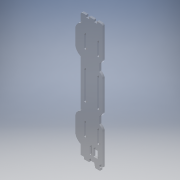
# Autodesk Inventor part: Left_wall
Saved by Autodesk Inventor 2016 (Build 200138000, 138)
## iProperties
Created: 2015-06-19
Part Number: Left_wall
Material: Generic
Document SubType Name: Modeling
Designer: Openlab
Density: 1 g/cm^3
Appearance: Polycarbonate - Clear
Author: Openlab
Autodesk Inventor part; units mm, degrees
ref_plane "YZ Plane" through (0, 0, 0) normal (1, 0, 0) x (0, 1, 0)
ref_plane "XZ Plane" through (0, 0, 0) normal (0, 1, 0) x (-1, 0, 0)
ref_plane "XY Plane" through (0, 0, 0) normal (0, 0, 1) x (1, 0, 0)
sketch "Sketch1" plane through (0, 0, 0) normal (0, 1, 0) x (-1, 0, 0)
  line L0 (26.5, -25) -> (23.5, -25)
  line L1 (26.5, -43) -> (23.5, -43)
  line L2 (26.5, -68) -> (23.5, -68)
  line L3 (26.5, -108) -> (23.5, -108)
  line L4 (8, -68) -> (5, -68)
  line L5 (8, -108) -> (5, -108)
  line L6 (8, -43) -> (5, -43)
  line L7 (8, -25) -> (5, -25)
  line L8 (23.5, -108) -> (23.5, -68)
  line L9 (23.5, -43) -> (23.5, -25)
  line L10 (8, -108) -> (8, -68)
  line L11 (8, -43) -> (8, -25)
  line L12 (8, -151) -> (8, -133)
  line L13 (26.5, -133) -> (23.5, -133)
  line L14 (8, -133) -> (5, -133)
  line L15 (23.5, -133) -> (23.5, -151)
  line L16 (23.5, -151) -> (26.5, -151)
  line L17 (5, -151) -> (8, -151)
  line L18 (18.5, -159) -> (16.7, -159)
  line L19 (16.7, -159) -> (16.7, -169)
  line L20 (16.7, -169) -> (18.5, -169)
  line L21 (18.5, -169) -> (18.5, -159)
  line L22 (15.75, -82) -> (15.75, -115) construction
  line L23 (13.2, -159) -> (7.2, -159)
  line L24 (7.2, -159) -> (7.2, -169)
  line L25 (7.2, -169) -> (13.2, -169)
  line L26 (13.2, -169) -> (13.2, -159)
  line L27 (26.5, -25) -> (26.5, -43)
  line L28 (26.5, -68) -> (26.5, -108)
  line L29 (26.5, -133) -> (26.5, -151)
  line L30 (5, -151) -> (5, -133)
  line L31 (5, -108) -> (5, -68)
  line L32 (5, -43) -> (5, -25)
  line L33 (12.25, -3) -> (8, -3)
  line L34 (19.25, -3) -> (19.25, 0)
  line L35 (19.25, 0) -> (12.25, 0)
  line L36 (12.25, 0) -> (12.25, -3)
  line L37 (19.25, -3) -> (23.5, -3)
  line L38 (5, -176) -> (5, -179)
  line L39 (12, -176) -> (19.5, -176)
  line L40 (19.5, -176) -> (19.5, -179)
  line L41 (19.5, -179) -> (26.2897, -179)
  line L42 (26.5, -176) -> (31.5, -176)
  line L43 (5, -179) -> (3.875, -179)
  line L44 (23.5, -3) -> (23.5, 0)
  line L45 (23.5, 0) -> (28.5, 0)
  line L46 (8, -3) -> (8, 0)
  line L47 (8, 0) -> (3, 0)
  line L48 (3.5, -180) -> (3.5, -181.5)
  line L49 (4, -182) -> (10.5533, -182)
  arc A0 (3.5, -181.5) -> (4, -182) centre (4, -181.5) ccw
  arc A1 (26.2897, -179) -> (26.5, -176) centre (5, -176) ccw
  arc A2 (5, -125.5838) -> (0, -133) centre (8, -133) ccw
  arc A3 (5, -60.5838) -> (0, -68) centre (8, -68) ccw
  line L50 (5, -50.4162) -> (5, -60.5838)
  line L51 (5, -115.4162) -> (5, -125.5838)
  line L52 (19.5, -120.5) -> (13.2, -120.5) construction
  arc A4 (0, -108) -> (5, -115.4162) centre (8, -108) ccw
  line L53 (0, -176) -> (0, -133)
  arc A5 (0, -43) -> (5, -50.4162) centre (8, -43) ccw
  line L54 (0, -108) -> (0, -68)
  line L55 (0, -43) -> (0, -3)
  arc A6 (31.5, -54.4564) -> (39, -43) centre (26.5, -43) ccw
  line L56 (39, -25) -> (39, -43)
  arc A7 (39, -25) -> (31.5, -13.5436) centre (26.5, -25) ccw
  line L57 (31.5, -3) -> (31.5, -13.5436)
  arc A8 (39, -133) -> (31.5, -121.5436) centre (26.5, -133) ccw
  line L58 (39, -151) -> (39, -133)
  arc A9 (31.5, -162.4564) -> (39, -151) centre (26.5, -151) ccw
  line L59 (31.5, -54.4564) -> (31.5, -121.5436)
  line L60 (31.5, -162.4564) -> (31.5, -176)
  line L61 (5, -176) -> (0, -176)
  line L62 (3.5, -180) -> (3.875, -179)
  line L63 (12, -176) -> (10.5533, -182)
  arc A10 (31.5, -3) -> (28.5, 0) centre (28.5, -3) ccw
  arc A11 (3, 0) -> (0, -3) centre (3, -3) ccw
  point P0 (0, 0)
  point P1 (3.5, -179)
  dimension "d7" = 18
  dimension "d8" = 25
  dimension "d9" = 40
  dimension "d39" = 18
  dimension "d43" = 1.8
  dimension "d45" = 10
  dimension "d51" = 3.5
  dimension "d52" = 6
  dimension "d56" = 3
  dimension "d61" = 25
  dimension "d62" = 15.5
  dimension "d63" = 22
  dimension "d64" = 25
  dimension "d65" = 7
  dimension "d74" = 173
  dimension "d75" = 15.5
  dimension "d80" = 3
  dimension "d81" = 1.5
  dimension "d82" = 7
  dimension "d85" = 7
  dimension "d90" = 5
  dimension "d92" = 25
  dimension "d94" = 13
  dimension "d97" = 1
  dimension "d98" = 0.5
  dimension "d100" = 7.5
  dimension "d101" = 7
  dimension "d102" = 5
  dimension "d103" = 7
  dimension "d104" = 6
  constraints: 129 end point, 24 collinear, 24 point on circle, 20 tangent, 15 point on line, 12 centre point, 10 perpendicular, 8 vertical, 7 coincident, 7 equal length, 5 horizontal, 5 parallel, 4 equal radius, 5 other
  measures "d7" distance between parallel lines of L1 L0
  measures "d8" distance between parallel lines of L2 L1
  measures "d9" distance between parallel lines of L3 L2
  measures "d39" distance of L13.end L15.end
  measures "d43" distance of L18.start L18.end
  measures "d45" distance of L20.end L18.start
  measures "d51" distance between parallel lines of L19 L26
  measures "d52" distance of L23.start L23.end
  measures "d56" distance of L0.start L0.end
  measures "d61" distance between parallel lines of L3 L13
  measures "d62" distance between parallel lines of L10 L8
  measures "d63" distance between parallel lines of L37 L0
  measures "d64" distance between parallel lines of L16 L42
  measures "d65" distance of L34.end L35.end
  measures "d74" distance between parallel lines of L42 L37
  measures "d75" distance between parallel lines of L46 L44
  measures "d80" distance between parallel lines of L49 L43
  measures "d81" distance between parallel lines of L48 L38
  measures "d82" distance between parallel lines of L39 L25
  measures "d85" distance from line of L42.start L40
  measures "d90" distance between parallel lines of L53 L30
  measures "d92" diameter of A6
  measures "d94" distance between parallel lines of L60 L21
  measures "d97" distance from line of L48.start L43
  measures "d98" radius of A0
  measures "d100" distance of L39.start L39.end
  measures "d101" distance from line of L38 L39.start
  measures "d102" distance from line of L60 L42.start
  measures "d103" angle of L63 L62
  measures "d104" diameter of A10
extrude "Extrusion3" add sketch "Sketch1" along normal blind 3
body "Solid3"
